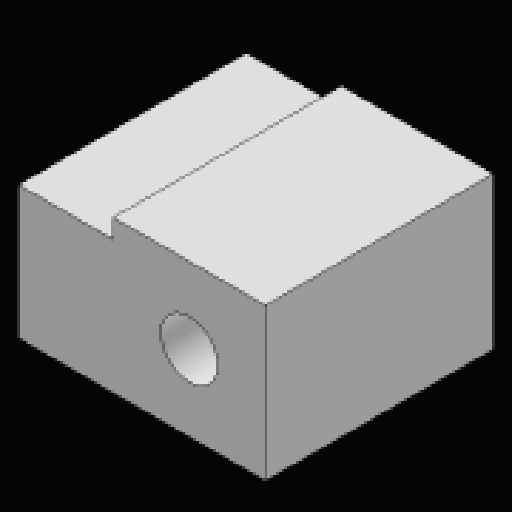
# Autodesk Inventor part: Rack
Saved by Autodesk Inventor 2023.2 (Build 272271030, 271C)
## iProperties
Created: 2023-11-11
Part Number: Rack
Material: Generic
Document SubType Name: Modeling
Designer: robpl
Density: 1 g/cm^3
Appearance: Default
Author: robpl
Autodesk Inventor part; units mm, degrees
ref_plane "YZ Plane" through (0, 0, 0) normal (1, 0, 0) x (0, 1, 0)
ref_plane "XZ Plane" through (0, 0, 0) normal (0, 1, 0) x (-1, 0, 0)
ref_plane "XY Plane" through (0, 0, 0) normal (0, 0, 1) x (1, 0, 0)
sketch "Sketch1" plane through (0, 0, 0) normal (0, 0, 1) x (1, 0, 0)
  line L0 (0, 0) -> (8, 0)
  line L1 (8, 0) -> (8, 8)
  line L2 (8, 8) -> (0, 8)
  line L3 (0, 8) -> (0, 0)
  line L4 (0, 0) -> (-8, 0)
  line L5 (-8, 0) -> (-8, 7)
  line L6 (-8, 7) -> (0, 7)
  line L7 (0, 7) -> (0, 0)
  point P0 (0, 7)
  dimension "d0" = 8
  dimension "d1" = 8
  dimension "d8" = 8
  dimension "d9" = 7
  constraints: 16 end point, 4 parallel, 2 horizontal, 2 perpendicular
  measures "d0" distance of L2.end L1.end
  measures "d1" distance of L1.end L0.end
  measures "d8" distance of L5.end L6.end
  measures "d9" distance of L4.end L5.end
extrude "Extrusion1" add sketch "Sketch1" along normal blind 12 contours L4 L5 L6 L3
sketch "Sketch2" plane through (0, 0, 12) normal (0, 0, 1) x (1, 0, 0)
  circle A0 centre (-4, 3.5) radius 2
  line L0 (0, 0) -> (0, 7) projected
  line L1 (0, 7) -> (-8, 7) projected
  line L2 (-8, 7) -> (-8, 0) projected
  line L3 (-8, 0) -> (0, 0) projected
  point P0 (-4, -1)
  point P1 (0, 3.5)
  point P2 (-4, 8)
  point P3 (-4, 0)
  point P4 (-8, 3.5)
  dimension "d4" = 4
  constraints: 3 vertical alignment, 2 horizontal alignment, 2 midpoint, 1 centre point
  measures "d4" diameter of A0
extrude "Extrusion2" cut sketch "Sketch2" against normal through all contours A0
body "Solid1"
